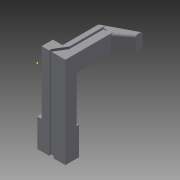
# Autodesk Inventor part: ConductiveThreadSide2
Saved by Autodesk Inventor 2015 (Build 190159000, 159)
## iProperties
Created: 2016-05-04
Part Number: ConductiveThreadSide2
Material: Generic
Document SubType Name: Modeling
Designer: Hatch
Density: 1 g/cm^3
Appearance: Default
Author: Hatch
Autodesk Inventor part; units mm, degrees
ref_plane "YZ Plane" through (0, 0, 0) normal (1, 0, 0) x (0, 1, 0)
ref_plane "XZ Plane" through (0, 0, 0) normal (0, 1, 0) x (-1, 0, 0)
ref_plane "XY Plane" through (0, 0, 0) normal (0, 0, 1) x (1, 0, 0)
sketch "Sketch1" plane through (0, 0, 0) normal (0, 1, 0) x (-1, 0, 0)
  line L0 (0, 0) -> (25, 0)
  line L1 (25, 0) -> (25, -81)
  line L2 (25, -81) -> (0, -81)
  line L3 (0, -81) -> (0, 0)
  dimension "d0" = 25
  dimension "d1" = 81
  constraints: 8 end point, 2 parallel, 1 horizontal, 1 perpendicular
  measures "d0" distance of L1.end L2.end
  measures "d1" distance of L0.end L1.end
extrude "Extrusion1" add sketch "Sketch1" along normal blind 25
sketch "Sketch2" plane through (0, 0, 0) normal (1, 0, 0) x (0, 0, -1)
  line L0 (81, 0) -> (81, 10)
  line L1 (81, 0) -> (81, 25) projected
  line L2 (81, 25) -> (21, 25)
  line L3 (21, 25) -> (21, 10)
  line L4 (21, 10) -> (81, 10)
  line L5 (81, 10) -> (81, 25)
  point P0 (0, 0)
  dimension "d4" = 10
  dimension "d5" = 60
  constraints: 10 end point, 2 parallel, 1 horizontal, 1 perpendicular, 1 point on line
  measures "d4" distance of L0.start L0.end
  measures "d5" distance of L4.end L3.end
extrude "Extrusion2" cut sketch "Sketch2" against normal through all
sketch "Sketch3" plane through (0, 10, -21) normal (0, 1, 0) x (1, 0, 0)
  line L0 (0, 60) -> (0, -21) projected
  line L1 (-25, 60) -> (0, 60)
  line L2 (0, 60) -> (0, 35)
  line L3 (0, 35) -> (-25, 35)
  line L4 (-25, 35) -> (-25, 60)
  circle A0 centre (-12.5, 47.5) radius 11.125
  dimension "d8" = 25
  dimension "d9" = 22.25
  constraints: 8 end point, 2 parallel, 1 centre point, 1 horizontal, 1 perpendicular, 1 point on line
  measures "d8" distance of L1.end L2.end
  measures "d9" diameter of A0
extrude "Extrusion3" cut sketch "Sketch3" against normal blind 7 contours A0
sketch "Sketch4" plane through (-25, 0, 0) normal (0, 0, 1) x (1, 0, 0)
  line L0 (25, 10) -> (0, 25)
  line L1 (0, 25) -> (25, 25)
  line L2 (0, 25) -> (25, 25) projected
  line L3 (25, 25) -> (25, 10)
  point P0 (25, 0)
  constraints: 6 end point, 1 collinear, 1 perpendicular
extrude "Extrusion4" cut sketch "Sketch4" against normal blind 21
sketch "Sketch5" plane through (0, 0, 0) normal (0, -1, 0) x (1, 0, 0)
  line L0 (0, 0) -> (-25, 0) projected
  line L1 (-10.5, -162) -> (-14.5, -162)
  line L2 (-14.5, -162) -> (-14.5, 0)
  line L3 (-14.5, 0) -> (-10.5, 0)
  line L4 (-10.5, 0) -> (-10.5, -162)
  line L5 (-25, -81) -> (0, -81) projected
  line L6 (-10.5, -162) -> (-14.5, 0) construction
  line L7 (-14.5, -162) -> (-10.5, 0) construction
  point P0 (-12.5, -81)
  dimension "d14" = 4
  constraints: 12 end point, 3 midpoint, 2 parallel, 1 horizontal, 1 perpendicular, 1 point on line
  measures "d14" distance of L2.end L3.end
extrude "Extrusion5" cut sketch "Sketch5" against normal blind 2
sketch "Sketch6" plane through (-25, 10, -81) normal (0, 1, 0) x (1, 0, 0)
  line L0 (25, -25) -> (0, -25)
  line L1 (0, -25) -> (0, 0)
  line L2 (0, 0) -> (25, 0)
  line L3 (25, 0) -> (25, -25)
  circle A0 centre (12.5, -12.5) radius 11.125 projected
  line L4 (25, -25) -> (0, 0) construction
  line L5 (0, -25) -> (25, 0) construction
  circle A1 centre (12.5, -12.5) radius 11.125
  point P0 (25, -81)
  constraints: 12 end point, 2 midpoint, 2 parallel, 1 centre point, 1 coincident, 1 concentric, 1 horizontal, 1 perpendicular
extrude "Extrusion6" add sketch "Sketch6" along normal blind 2
sketch "Sketch7" plane through (-12.5, 3, -68.5) normal (0, 1, 0) x (1, 0, 0)
  circle A0 centre (0, 0) radius 11.125 projected
  circle A1 centre (0, 0) radius 11.125
  point P0 (12.5, -68.5)
  constraints: 1 centre point, 1 coincident
extrude "Extrusion7" add sketch "Sketch7" along normal blind 2
sketch "Sketch8" plane through (-25, 0, 0) normal (0, 0, 1) x (1, 0, 0)
  line L0 (0, 0) -> (0, 50)
  line L1 (0, 50) -> (25, 50)
  line L2 (25, 50) -> (25, 37)
  line L3 (25, 37) -> (0, 50)
  line L4 (25, 37) -> (25, 10)
  line L5 (25, 0) -> (25, 12) projected
  line L6 (25, 10) -> (0, 25)
  line L7 (25, 10) -> (0, 25) projected
  line L8 (0, 50) -> (0, 25)
  line L9 (25, 10) -> (0, 25)
  line L10 (25, 37) -> (25, 10)
  line L11 (25, 10) -> (0, 10) projected
  line L12 (25, 37) -> (0, 50)
  dimension "d21" = 50
  dimension "d22" = 13
  constraints: 20 end point, 4 collinear, 2 perpendicular, 2 vertical, 1 horizontal
  measures "d21" distance of L0.start L0.end
  measures "d22" distance of L1.end L2.end
extrude "Extrusion8" add sketch "Sketch8" against normal blind 15 contours L0 L3 L4 L6
sketch "Sketch9" plane through (-25, 0, -81) normal (-1, 0, 0) x (0, 0, 1)
  line L0 (66, 25) -> (60, 25)
  line L1 (60, 25) -> (60, 10)
  line L2 (60, 10) -> (66, 10)
  line L3 (66, 10) -> (66, 25)
  point P0 (81, 0)
  constraints: 8 end point, 2 parallel, 1 horizontal, 1 perpendicular
extrude "Extrusion9" cut sketch "Sketch9" against normal through all
sketch "Sketch10" plane through (-25, 0, -15) normal (0, 0, -1) x (-1, 0, 0)
  point P0 (-25, 0)
sketch "Sketch11" plane through (-10.5, 0, 0) normal (0, 0, 1) x (1, 0, 0)
  line L0 (10.5, 10) -> (-2, 10)
  line L1 (-2, 10) -> (-2, 47.9639)
  line L2 (-2, 47.9639) -> (10.5, 47.9639)
  line L3 (10.5, 47.9639) -> (10.5, 10)
  point P0 (10.5, 0)
  constraints: 8 end point, 2 parallel, 1 horizontal, 1 perpendicular
extrude "Extrusion10" cut sketch "Sketch11" against normal blind 15
sketch "Sketch12" plane through (0, 0, 0) normal (0, 0, 1) x (1, 0, 0)
  line L0 (-12.5, 43.5) -> (-37.3421, 56.4179)
  line L1 (-25, 50) -> (-12.5, 43.5) projected
  line L2 (-37.3421, 56.4179) -> (-37.3421, 50)
  line L3 (-37.3421, 50) -> (-25, 40.4241)
  line L4 (-25, 0) -> (-25, 50) projected
  line L5 (-12.5, 43.5) -> (-25, 40.4241)
  point P0 (0, 0)
  dimension "d29" = 28
  constraints: 8 end point, 1 collinear, 1 point on line, 1 vertical
  measures "d29" distance of L0.start L0.end
extrude "Extrusion11" add sketch "Sketch12" against normal blind 15 contours L4 L3 L2 L0
fillet "Fillet1" radius 2 1 edges at (-24.921, 49.9589, 0)
fillet "Fillet2" radius 2 1 edges at (-31.171, 45.212, 0)
fillet "Fillet3" radius 2 2 edges at (-24.921, 49.9589, -15) (-31.171, 45.212, -15)
sketch "Sketch13" plane through (0, 0, 0) normal (0, 0, 1) x (1, 0, 0)
  line L0 (-10.5, 2) -> (-16.5509, 12)
  line L1 (-23.625, 12) -> (-1.375, 12) projected
  line L2 (-16.5509, 12) -> (-16.5509, 42.153)
  line L3 (-16.5509, 42.153) -> (-20.5509, 42.153)
  line L4 (-20.5509, 42.153) -> (-20.5509, 12)
  line L5 (-20.5509, 12) -> (-14.5, 2)
  line L6 (-14.5, 2) -> (-10.5, 2)
  line L7 (-14.5, 2) -> (-10.5, 2) projected
  point P0 (0, 0)
  dimension "d35" = 4
  constraints: 12 end point, 2 point on line, 1 collinear, 1 horizontal, 1 perpendicular, 1 vertical
  measures "d35" distance of L2.end L3.end
extrude "Extrusion12" cut sketch "Sketch13" against normal blind 2
fillet "Fillet4" radius 2 1 edges at (-18.5509, 42.153, 0)
sketch "Sketch14" plane through (0, 10, 0) normal (0, 1, 0) x (1, 0, 0)
  line L0 (0, 56) -> (-25, 56) projected
  line L1 (0, 0) -> (-4, 0)
  line L2 (-4, 0) -> (-4, 56)
  line L3 (-4, 56) -> (0, 56)
  line L4 (0, 56) -> (0, 0)
  dimension "d39" = 4
  constraints: 8 end point, 2 parallel, 1 horizontal, 1 perpendicular, 1 point on line
  measures "d39" distance of L2.end L3.end
extrude "Extrusion13" cut sketch "Sketch14" against normal through all
sketch "Sketch15" plane through (-25, 0, -15) normal (0, 0, -1) x (-1, 0, 0)
  point P0 (-25, 0)
mirror "Mirror1" about plane through (0, 0, 0) normal (1, 0, 0)
sketch "Sketch16" plane through (0, 0, 0) normal (0, -1, 0) x (1, 0, 0)
  line L0 (-10.5, -81) -> (10.5, -81) projected
  line L1 (0, -81) -> (-50.0267, -81)
  line L2 (-50.0267, -81) -> (-50.0267, 5.7652)
  line L3 (-50.0267, 5.7652) -> (0, 5.7652)
  line L4 (0, 5.7652) -> (0, -81)
  point P0 (0, 0)
  constraints: 8 end point, 2 parallel, 1 horizontal, 1 midpoint, 1 perpendicular
extrude "Extrusion14" cut sketch "Sketch16" against normal through all
body "Solid1"
